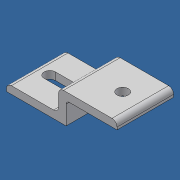
# Autodesk Inventor part: 093P45LN Bracket
Saved by Autodesk Inventor 2012 (Build 160160000, 160)
## iProperties
Created: 2014-06-11
Part Number: 093P45LN Bracket
Material: Aluminum-6061
Document SubType Name: Modeling
Designer: Mike Taylor
Mass: 71.8175 g
Surface Area: 109.095 cm^2
Volume: 26.5009 cm^3
Density: 2.71 g/cm^3
Author: Mike Taylor
Autodesk Inventor part; units mm, degrees
ref_plane "YZ Plane" through (0, 0, 0) normal (1, 0, 0) x (0, 1, 0)
ref_plane "XZ Plane" through (0, 0, 0) normal (0, 1, 0) x (-1, 0, 0)
ref_plane "XY Plane" through (0, 0, 0) normal (0, 0, 1) x (1, 0, 0)
sketch "Sketch1" plane through (0, 0, 0) normal (0, 0, 1) x (1, 0, 0)
  line L0 (0, 0) -> (0, 6)
  line L1 (0, 6) -> (41.5, 6)
  line L2 (41.5, 6) -> (41.5, 23.5)
  line L3 (41.5, 23.5) -> (88, 23.5)
  line L4 (88, 23.5) -> (88, 17.5)
  line L5 (88, 17.5) -> (47.5, 17.5)
  line L6 (47.5, 17.5) -> (47.5, 0)
  line L7 (47.5, 0) -> (0, 0)
  dimension "d0" = 6
  dimension "d1" = 6
  dimension "d2" = 6
  dimension "d3" = 88
  dimension "d4" = 41.5
  dimension "d5" = 17.5
  constraints: 16 end point, 6 parallel, 1 perpendicular, 1 vertical
  measures "d0" distance between parallel lines of L3 L5
  measures "d1" distance between parallel lines of L7 L1
  measures "d2" distance between parallel lines of L2 L6
  measures "d3" distance between parallel lines of L0 L4
  measures "d4" distance between parallel lines of L0 L2
  measures "d5" distance between parallel lines of L1 L3
extrude "Extrusion1" add sketch "Sketch1" along normal blind 45
sketch "Sketch3" plane through (88, 17.5, 0) normal (0, -1, 0) x (1, 0, 0)
  line L0 (0, 0) -> (-40.5, 0) projected
  line L1 (-40.5, 0) -> (-40.5, 45) projected
  point P0 (-38, 0)
  point P1 (-88, 0)
  point P2 (-17.9956, 22.5044)
  dimension "d9" = 22.5044
  dimension "d10" = 22.5044
  measures "d9" distance from line of L1 point (-17.996, 22.504)
  measures "d10" distance from line of L0 point (-17.996, 22.504)
hole "Hole1" at (70.0044, 17.5, 22.5044) direction (0, 1, 0) diameter 9 end through all
sketch "Sketch4" plane through (0, 0, 0) normal (0, -1, 0) x (1, 0, 0)
  line L0 (47.5, 45) -> (0, 45) projected
  line L1 (47.5, 0) -> (47.5, 45) projected
  circle A0 centre (30, 22.4956) radius 4.5
  circle A1 centre (12, 22.4956) radius 4.5
  line L2 (30, 17.9956) -> (12, 17.9956)
  line L3 (12, 26.9956) -> (30, 26.9956)
  dimension "d18" = 17.5
  dimension "d19" = 18
  dimension "d20" = 22.5044
  dimension "d21" = 9
  dimension "d22" = 9
  constraints: 4 end point, 4 point on circle, 2 centre point, 2 coincident, 2 tangent, 1 horizontal alignment, 1 parallel
  measures "d18" distance from line of L1 point (30, 22.496)
  measures "d19" distance of point (30, 22.496) point (12, 22.496)
  measures "d20" distance from line of point (12, 22.496) L0
  measures "d21" diameter of A1
  measures "d22" diameter of A0
extrude "Extrusion2" cut sketch "Sketch4" against normal blind 45
fillet "Fillet2" radius 2.5 1 edges at (47.5, 17.5, 22.5)
fillet "Fillet3" radius 4 4 edges at (88, 23.5, 22.5) (41.5, 23.5, 22.5) (0, 6, 22.5) (41.5, 6, 22.5)
equation "\"d1\" = d0"
equation "\"d2\" = d0"
equation "\"d22\" = d21"
body "Solid1"
